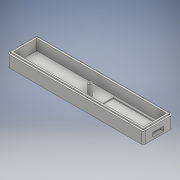
# Autodesk Inventor part: Base Wide
Saved by Autodesk Inventor 2018 (Build 220112000, 112)
## iProperties
Created: 2018-05-10
Part Number: Base Wide
Material: Generic
Document SubType Name: Modeling
Designer: mtsti
Density: 1 g/cm^3
Appearance: Default
Author: mtsti
Autodesk Inventor part; units mm, degrees
sketch "Sketch1" plane through (0, 0, 0) normal (0, 0, 1) x (1, 0, 0)
  line L0 (0, 0) -> (128, 0)
  line L1 (128, 0) -> (128, 28)
  line L2 (128, 28) -> (0, 28)
  line L3 (0, 28) -> (0, 0)
  dimension "d57" = 128
  dimension "d58" = 28
  constraints: 8 end point, 2 parallel, 1 horizontal, 1 perpendicular
  measures "d57" distance of L2.end L1.end
  measures "d58" distance of L1.end L0.end
ref_plane "Work Plane7" through (0, 0, 12) normal (0, 0, 1) x (1, 0, 0)
sketch "Sketch2" plane through (0, 0, 12) normal (0, 0, 1) x (1, 0, 0)
  line L0 (3, 3) -> (85, 3)
  line L1 (85, 3) -> (85, 45)
  line L2 (85, 45) -> (3, 45)
  line L3 (3, 45) -> (3, 3)
  line L4 (88, 48) -> (0, 48) projected
  line L5 (88, 0) -> (88, 48) projected
  line L6 (0, 0) -> (88, 0) projected
  line L7 (0, 48) -> (0, 0) projected
  dimension "d4" = 3
  dimension "d5" = 3
  dimension "d6" = 3
  dimension "d7" = 3
  constraints: 8 end point, 2 parallel, 1 horizontal, 1 perpendicular
  measures "d4" distance between parallel lines of L4 L2
  measures "d5" distance between parallel lines of L5 L1
  measures "d6" distance between parallel lines of L6 L0
  measures "d7" distance between parallel lines of L7 L3
ref_plane "Work Plane6" through (0, 0, 12) normal (0, 0, 1) x (1, 0, 0)
sketch "Sketch3" plane through (0, 0, 12) normal (0, 0, 1) x (1, 0, 0)
  line L0 (1.5, 46.5) -> (86.5, 46.5)
  line L1 (86.5, 46.5) -> (86.5, 1.5)
  line L2 (86.5, 1.5) -> (1.5, 1.5)
  line L3 (1.5, 1.5) -> (1.5, 46.5)
  line L4 (0, 0) -> (88, 0) projected
  line L5 (0, 48) -> (0, 0) projected
  line L6 (88, 0) -> (0, 0)
  line L7 (0, 0) -> (0, 48)
  line L8 (0, 48) -> (88, 48)
  line L9 (88, 48) -> (88, 0)
  dimension "d10" = 1.5
  dimension "d11" = 1.5
  dimension "d12" = 1.5
  dimension "d13" = 1.5
  constraints: 16 end point, 4 parallel, 2 horizontal, 2 perpendicular
  measures "d10" distance between parallel lines of L8 L0
  measures "d11" distance between parallel lines of L5 L3
  measures "d12" distance between parallel lines of L4 L2
  measures "d13" distance between parallel lines of L9 L1
ref_plane "Work Plane5" through (0, 0, 12) normal (0, 0, 1) x (1, 0, 0)
sketch "Sketch4" plane through (0, 0, 12) normal (0, 0, 1) x (1, 0, 0)
  circle A0 centre (5.5, 24) radius 1
  circle A1 centre (82.5, 24) radius 1
  line L0 (3, 45) -> (85, 45) projected
  line L1 (3, 3) -> (3, 45) projected
  line L2 (3, 25.5) -> (5.5, 25.5)
  line L3 (5.5, 25.5) -> (5.5, 22.5)
  line L4 (5.5, 22.5) -> (3, 22.5)
  line L5 (3, 22.5) -> (3, 25.5)
  circle A2 centre (5.5, 24) radius 1.5
  line L6 (85, 45) -> (85, 3) projected
  line L7 (85, 22.5) -> (82.5, 22.5)
  line L8 (82.5, 22.5) -> (82.5, 25.5)
  line L9 (82.5, 25.5) -> (85, 25.5)
  line L10 (85, 25.5) -> (85, 22.5)
  circle A3 centre (82.5, 24) radius 1.5
  point P0 (0, 0)
  dimension "d17" = 2
  dimension "d18" = 2
  dimension "d19" = 21
  dimension "d20" = 21
  dimension "d21" = 2.5
  dimension "d22" = 3
  dimension "d23" = 1.5
  dimension "d24" = 2.5
  dimension "d25" = 2.5
  dimension "d26" = 3
  dimension "d27" = 1.5
  constraints: 16 end point, 4 parallel, 2 centre point, 2 coincident, 2 horizontal, 2 perpendicular, 2 point on line, 2 vertical alignment, 4 other
  measures "d17" diameter of A0
  measures "d18" diameter of A1
  measures "d19" distance from line of A0.centre L0
  measures "d20" distance from line of A1.centre L0
  measures "d21" distance from line of A0.centre L1
  measures "d22" distance of L2.end L3.end
  measures "d23" distance from line of L4 A0.centre
  measures "d24" distance from line of L6 A1.centre
  measures "d25" distance of L8.end L9.end
  measures "d26" distance of L7.end L8.end
  measures "d27" distance from line of A1.centre L9
ref_plane "Work Plane4" through (0, 0, 12) normal (0, 0, 1) x (1, 0, 0)
sketch "Sketch5" plane through (0, 0, 12) normal (0, 0, 1) x (1, 0, 0)
  circle A0 centre (5.5, 24) radius 1
  circle A1 centre (82.5, 24) radius 1
  line L0 (3, 25.5) -> (3, 22.5) projected
  line L1 (3, 22.5) -> (5.5, 22.5) projected
  line L2 (82.5, 22.5) -> (85, 22.5) projected
  line L3 (85, 22.5) -> (85, 25.5) projected
  point P0 (0, 0)
  dimension "d30" = 2
  dimension "d31" = 2
  dimension "d32" = 2.5
  dimension "d33" = 1.5
  dimension "d34" = 1.5
  dimension "d35" = 2.5
  constraints: 2 centre point
  measures "d30" diameter of A0
  measures "d31" diameter of A1
  measures "d32" distance from line of A0.centre L0
  measures "d33" distance from line of L1 A0.centre
  measures "d34" distance from line of L2 A1.centre
  measures "d35" distance from line of A1.centre L3
ref_plane "Work Plane1" through (0, 0, 3) normal (0, 0, 1) x (1, 0, 0)
sketch "Sketch6" plane through (0, 0, 3) normal (0, 0, 1) x (1, 0, 0)
  line L0 (35, 45) -> (53, 45)
  line L1 (53, 45) -> (53, 9)
  line L2 (53, 9) -> (35, 9)
  line L3 (35, 9) -> (35, 45)
  line L4 (3, 45) -> (85, 45) projected
  line L5 (3, 3) -> (3, 45) projected
  point P0 (0, 0)
  point P1 (3, 25.5)
  dimension "d38" = 18
  dimension "d39" = 36
  dimension "d40" = 0
  dimension "d41" = 32
  dimension "d50" = 82
  constraints: 8 end point, 2 parallel, 1 horizontal, 1 perpendicular
  measures "d38" distance of L1.end L2.end
  measures "d39" distance of L0.end L1.end
  measures "d40" distance between parallel lines of L4 L0
  measures "d41" distance between parallel lines of L3 L5
  measures "d50" distance of L4.start L4.end
ref_plane "Work Plane2" through (0, 48, 11) normal (0, 1, 0) x (1, 0, 0)
sketch "Sketch7" plane through (0, 48, 11) normal (0, 1, 0) x (1, 0, 0)
  line L0 (48.5, 4.8) -> (40.5, 4.8)
  line L1 (40.5, 4.8) -> (40.5, 8)
  line L2 (40.5, 8) -> (48.5, 8)
  line L3 (48.5, 8) -> (48.5, 4.8)
  line L4 (88, 11) -> (0, 11) projected
  line L5 (86, 11) -> (86, 0) projected
  dimension "d44" = 8
  dimension "d45" = 3.2
  dimension "d46" = 3
  dimension "d47" = 37.5
  constraints: 8 end point, 2 parallel, 1 horizontal, 1 perpendicular
  measures "d44" distance of L1.end L2.end
  measures "d45" distance of L0.end L1.end
  measures "d46" distance between parallel lines of L4 L2
  measures "d47" distance between parallel lines of L5 L3
ref_plane "Work Plane3" through (0, 48, 11) normal (0, 1, 0) x (1, 0, 0)
sketch "Sketch8" plane through (0, 48, 11) normal (0, 1, 0) x (1, 0, 0)
  line L0 (50.5, 9.5) -> (38.5, 9.5)
  line L1 (38.5, 9.5) -> (38.5, 3.3)
  line L2 (38.5, 3.3) -> (50.5, 3.3)
  line L3 (50.5, 3.3) -> (50.5, 9.5)
  line L4 (48.5, 8) -> (48.5, 4.8) projected
  line L5 (40.5, 4.8) -> (40.5, 8) projected
  line L6 (48.5, 4.8) -> (40.5, 4.8) projected
  line L7 (40.5, 8) -> (48.5, 8) projected
  point P0 (0, 11)
  dimension "d51" = 2
  dimension "d52" = 2
  dimension "d53" = 1.5
  dimension "d54" = 1.5
  constraints: 8 end point, 2 parallel, 1 horizontal, 1 perpendicular
  measures "d51" distance between parallel lines of L3 L4
  measures "d52" distance between parallel lines of L1 L5
  measures "d53" distance between parallel lines of L2 L6
  measures "d54" distance between parallel lines of L7 L0
extrude "Extrusion9" add sketch "Sketch1" along normal blind 11
sketch "Sketch9" plane through (0, 0, 11) normal (0, 0, 1) x (1, 0, 0)
  line L0 (3, 3) -> (125, 3)
  line L1 (125, 3) -> (125, 25)
  line L2 (125, 25) -> (3, 25)
  line L3 (3, 25) -> (3, 3)
  line L4 (0, 0) -> (128, 0) projected
  line L5 (0, 28) -> (0, 0) projected
  dimension "d61" = 122
  dimension "d62" = 22
  dimension "d63" = 3
  dimension "d64" = 3
  constraints: 8 end point, 2 parallel, 1 horizontal, 1 perpendicular
  measures "d61" distance of L2.end L1.end
  measures "d62" distance of L2.end L0.start
  measures "d63" distance between parallel lines of L4 L0
  measures "d64" distance between parallel lines of L5 L3
extrude "Extrusion10" cut sketch "Sketch9" against normal blind 9
fillet "Fillet2" radius 2 4 edges at (128, 0, 5.5) (0, 28, 5.5) (0, 0, 5.5) (128, 28, 5.5)
sketch "Sketch10" plane through (0, 0, 11) normal (0, 0, 1) x (1, 0, 0)
  line L0 (3, 3) -> (3, 25) projected
  line L1 (125, 25) -> (125, 3) projected
  line L2 (3, 25) -> (125, 25)
  line L3 (125, 25) -> (125, 3)
  line L4 (125, 3) -> (3, 3)
  line L5 (3, 3) -> (3, 25)
  line L6 (1.5, 26.5) -> (126.5, 26.5)
  line L7 (126.5, 26.5) -> (126.5, 1.5)
  line L8 (126.5, 1.5) -> (1.5, 1.5)
  line L9 (1.5, 1.5) -> (1.5, 26.5)
  point P0 (0, 0)
  dimension "d69" = 1.5
  dimension "d70" = 1.5
  dimension "d71" = 1.5
  dimension "d72" = 1.5
  constraints: 16 end point, 4 parallel, 2 horizontal, 2 perpendicular
  measures "d69" distance between parallel lines of L2 L6
  measures "d70" distance between parallel lines of L0 L9
  measures "d71" distance between parallel lines of L4 L8
  measures "d72" distance between parallel lines of L1 L7
extrude "Extrusion11" add sketch "Sketch10" along normal blind 1
sketch "Sketch11" plane through (0, 0, 2) normal (0, 0, 1) x (1, 0, 0)
  line L0 (125, 5.15) -> (77, 5.15)
  line L1 (77, 5.15) -> (77, 22.85)
  line L2 (77, 22.85) -> (125, 22.85)
  line L3 (125, 22.85) -> (125, 5.15)
  line L4 (125, 25) -> (125, 3) projected
  line L5 (3, 25) -> (125, 25) projected
  point P0 (0, 0)
  dimension "d75" = 48
  dimension "d76" = 17.7
  dimension "d77" = 0
  dimension "d78" = 2.15
  constraints: 8 end point, 2 parallel, 1 horizontal, 1 perpendicular
  measures "d75" distance of L1.end L2.end
  measures "d76" distance of L0.end L1.end
  measures "d77" distance between parallel lines of L4 L3
  measures "d78" distance between parallel lines of L5 L2
extrude "Extrusion12" cut sketch "Sketch11" against normal blind 1
sketch "Sketch13" plane through (128, 2, 0) normal (1, 0, 0) x (0, 0, -1)
  line L0 (-2, 7) -> (-6, 7)
  line L1 (-6, 7) -> (-6, 17)
  line L2 (-6, 17) -> (-2, 17)
  line L3 (-2, 17) -> (-2, 7)
  line L4 (-11, -2) -> (0, -2) projected
  line L5 (0, 0) -> (0, 24) projected
  dimension "d81" = 4
  dimension "d82" = 10
  dimension "d83" = 9
  dimension "d84" = 2
  constraints: 8 end point, 2 parallel, 1 horizontal, 1 perpendicular
  measures "d81" distance of L1.end L2.end
  measures "d82" distance of L0.end L1.end
  measures "d83" distance between parallel lines of L4 L0
  measures "d84" distance between parallel lines of L5 L3
extrude "Extrusion13" cut sketch "Sketch13" against normal blind 3
sketch "Sketch14" plane through (0, 0, 2) normal (0, 0, 1) x (1, 0, 0)
  circle A0 centre (64, 14) radius 1
  circle A1 centre (64, 14) radius 2
  line L0 (3, 25) -> (125, 25) projected
  line L1 (3, 3) -> (3, 25) projected
  point P0 (0, 0)
  dimension "d87" = 2
  dimension "d88" = 4
  dimension "d89" = 11
  dimension "d90" = 61
  constraints: 2 centre point, 1 coincident
  measures "d87" diameter of A0
  measures "d88" diameter of A1
  measures "d89" distance from line of A0.centre L0
  measures "d90" distance from line of A0.centre L1
extrude "Extrusion14" add sketch "Sketch14" along normal blind 10
body "Solid2"
